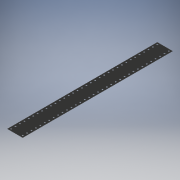
# Autodesk Inventor part: Foam NPS 18
Saved by Autodesk Inventor 2019 (Build 230136000, 136)
## iProperties
Created: 2016-08-30
Part Number: Foam NPS 18
Material: Rubber, Silicone
Document SubType Name: Modeling
Designer: IEUser
Density: 1.25 g/cm^3
Appearance: Rubber - Black
Author: IEUser
Autodesk Inventor part; units mm, degrees
ref_plane "YZ Plane" through (0, 0, 0) normal (1, 0, 0) x (0, 1, 0)
ref_plane "XZ Plane" through (0, 0, 0) normal (0, 1, 0) x (-1, 0, 0)
ref_plane "XY Plane" through (0, 0, 0) normal (0, 0, 1) x (1, 0, 0)
sketch "Foam Scheme" plane through (0, 0, 0) normal (0, 1, 0) x (-1, 0, 0)
  line L0 (929.5, -94) -> (-929.5, -94)
  line L1 (-929.5, -94) -> (-929.5, 94)
  line L2 (-929.5, 94) -> (929.5, 94)
  line L3 (929.5, 94) -> (929.5, -94)
  circle A0 centre (907.5, -72) radius 9.5
  circle A1 centre (852.5, -72) radius 9.5
  circle A2 centre (797.5, -72) radius 9.5
  circle A3 centre (742.5, -72) radius 9.5
  circle A4 centre (687.5, -72) radius 9.5
  circle A5 centre (632.5, -72) radius 9.5
  circle A6 centre (577.5, -72) radius 9.5
  circle A7 centre (522.5, -72) radius 9.5
  circle A8 centre (467.5, -72) radius 9.5
  circle A9 centre (412.5, -72) radius 9.5
  circle A10 centre (357.5, -72) radius 9.5
  circle A11 centre (302.5, -72) radius 9.5
  circle A12 centre (247.5, -72) radius 9.5
  circle A13 centre (192.5, -72) radius 9.5
  circle A14 centre (137.5, -72) radius 9.5
  circle A15 centre (82.5, -72) radius 9.5
  circle A16 centre (27.5, -72) radius 9.5
  circle A17 centre (-27.5, -72) radius 9.5
  circle A18 centre (907.5, 72) radius 9.5
  circle A19 centre (852.5, 72) radius 9.5
  circle A20 centre (797.5, 72) radius 9.5
  circle A21 centre (742.5, 72) radius 9.5
  circle A22 centre (687.5, 72) radius 9.5
  circle A23 centre (632.5, 72) radius 9.5
  circle A24 centre (577.5, 72) radius 9.5
  circle A25 centre (522.5, 72) radius 9.5
  circle A26 centre (467.5, 72) radius 9.5
  circle A27 centre (412.5, 72) radius 9.5
  circle A28 centre (357.5, 72) radius 9.5
  circle A29 centre (302.5, 72) radius 9.5
  circle A30 centre (247.5, 72) radius 9.5
  circle A31 centre (192.5, 72) radius 9.5
  circle A32 centre (137.5, 72) radius 9.5
  circle A33 centre (82.5, 72) radius 9.5
  circle A34 centre (27.5, 72) radius 9.5
  circle A35 centre (-27.5, 72) radius 9.5
  circle A36 centre (-82.5, -72) radius 9.5
  circle A37 centre (-82.5, 72) radius 9.5
  circle A38 centre (-137.5, -72) radius 9.5
  circle A39 centre (-137.5, 72) radius 9.5
  circle A40 centre (-192.5, -72) radius 9.5
  circle A41 centre (-192.5, 72) radius 9.5
  circle A42 centre (-247.5, -72) radius 9.5
  circle A43 centre (-247.5, 72) radius 9.5
  circle A44 centre (-302.5, -72) radius 9.5
  circle A45 centre (-302.5, 72) radius 9.5
  circle A46 centre (-357.5, -72) radius 9.5
  circle A47 centre (-357.5, 72) radius 9.5
  circle A48 centre (-412.5, -72) radius 9.5
  circle A49 centre (-412.5, 72) radius 9.5
  circle A50 centre (-467.5, -72) radius 9.5
  circle A51 centre (-467.5, 72) radius 9.5
  circle A52 centre (-522.5, -72) radius 9.5
  circle A53 centre (-522.5, 72) radius 9.5
  circle A54 centre (-577.5, -72) radius 9.5
  circle A55 centre (-577.5, 72) radius 9.5
  circle A56 centre (-632.5, -72) radius 9.5
  circle A57 centre (-632.5, 72) radius 9.5
  circle A58 centre (-687.5, -72) radius 9.5
  circle A59 centre (-687.5, 72) radius 9.5
  circle A60 centre (-742.5, -72) radius 9.5
  circle A61 centre (-742.5, 72) radius 9.5
  circle A62 centre (-797.5, -72) radius 9.5
  circle A63 centre (-797.5, 72) radius 9.5
  circle A64 centre (-852.5, -72) radius 9.5
  circle A65 centre (-852.5, 72) radius 9.5
  circle A66 centre (-907.5, -72) radius 9.5
  circle A67 centre (-907.5, 72) radius 9.5
  point P0 (0, 0)
  dimension "d0" = 1859
  dimension "d1" = 929.5
  dimension "d2" = 188
  dimension "d3" = 94
  dimension "d4" = 19
  dimension "d5" = 22
  dimension "d6" = 22
  dimension "d9" = 55
  dimension "d12" = 144
  constraints: 68 centre point, 8 end point, 2 horizontal, 2 parallel, 1 perpendicular, 1 vertical, 134 other
  measures "d0" distance of L0.start L0.end
  measures "d1" distance from line of point (0, 0) L3
  measures "d2" distance of L2.end L0.start
  measures "d3" distance from line of point (0, 0) L0
  measures "d4" diameter of A0
  measures "d5" distance from line of L3 A0.centre
  measures "d6" distance from line of L0 A0.centre
  measures "d9" distance of A0.centre A1.centre
  measures "d12" distance of A0.centre A18.centre
extrude "Foam Body" add sketch "Foam Scheme" along normal blind 1.5
equation "\"d1\" = 0.5 * d0"
equation "\"d3\" = 0.5 * d2"
body "Solid2"
